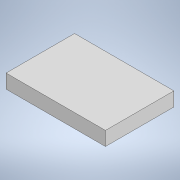
# Autodesk Inventor part: Battery
Saved by Autodesk Inventor 2020 (Build 240168000, 168)
## iProperties
Created: 2019-07-11
Part Number: Battery
Material: Generic
Document SubType Name: Modeling
Designer: tyrre
Density: 1 g/cm^3
Appearance: Default
Author: tyrre
Autodesk Inventor part; units mm, degrees
ref_plane "YZ Plane" through (0, 0, 0) normal (1, 0, 0) x (0, 1, 0)
ref_plane "XZ Plane" through (0, 0, 0) normal (0, 1, 0) x (-1, 0, 0)
ref_plane "XY Plane" through (0, 0, 0) normal (0, 0, 1) x (1, 0, 0)
sketch "Sketch1" plane through (0, 0, 0) normal (0, 0, 1) x (1, 0, 0)
  line L0 (-18.5, -2.6) -> (18.5, -2.6)
  line L1 (18.5, -2.6) -> (18.5, 2.6)
  line L2 (18.5, 2.6) -> (-18.5, 2.6)
  line L3 (-18.5, 2.6) -> (-18.5, -2.6)
  line L4 (-18.5, -2.6) -> (18.5, 2.6) construction
  line L5 (18.5, -2.6) -> (-18.5, 2.6) construction
  point P0 (0, 0)
  dimension "d0" = 37
  dimension "d1" = 5.2
  constraints: 12 end point, 2 midpoint, 2 parallel, 1 horizontal, 1 perpendicular
  measures "d0" distance of L2.end L1.end
  measures "d1" distance of L1.end L0.end
extrude "Extrusion1" add sketch "Sketch1" along normal mid plane 25.5
body "Solid1"
